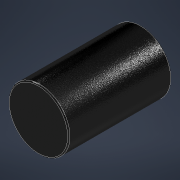
# Autodesk Inventor part: 05_Bloczek
Saved by Autodesk Inventor 2022 (Build 260153000, 153)
## iProperties
Created: 2022-05-07
Part Number: 05_Bloczek
Material: Generic
Document SubType Name: Modeling
Designer: pzach
Density: 1 g/cm^3
Appearance: Black
Author: pzach
Autodesk Inventor part; units mm, degrees
ref_plane "YZ Plane" through (0, 0, 0) normal (1, 0, 0) x (0, 1, 0)
ref_plane "XZ Plane" through (0, 0, 0) normal (0, 1, 0) x (-1, 0, 0)
ref_plane "XY Plane" through (0, 0, 0) normal (0, 0, 1) x (1, 0, 0)
sketch "Sketch1" plane through (0, 0, 0) normal (0, 0, 1) x (1, 0, 0)
  circle A0 centre (0, 0) radius 530
  dimension "d0" = 1060
  constraints: 1 centre point, 1 coincident
  measures "d0" diameter of A0
extrude "Extrusion1" add sketch "Sketch1" along normal blind 1800
fillet "Fillet1" radius 20 2 edges at (-530, 0, 1800) (-530, 0, 0)
body "Solid1"
